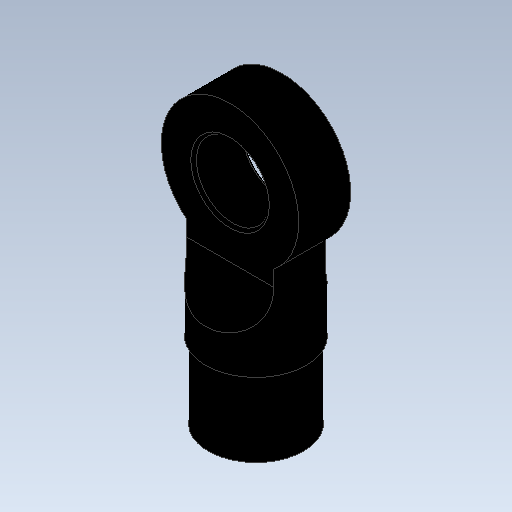
# Autodesk Inventor part: Conexion_superioript
Saved by Autodesk Inventor 2020 (Build 240168000, 168)
## iProperties
Created: 2019-09-21
Part Number: Conexion_superioript
Material: Plástico ABS
Document SubType Name: Modeling
Designer: axelj
Density: 1.06 g/cm^3
Appearance: Anodizado - Negro
Author: axelj
Autodesk Inventor part; units mm, degrees
ref_plane "YZ Plane" through (0, 0, 0) normal (1, 0, 0) x (0, 1, 0)
ref_plane "XZ Plane" through (0, 0, 0) normal (0, 1, 0) x (-1, 0, 0)
ref_plane "XY Plane" through (0, 0, 0) normal (0, 0, 1) x (1, 0, 0)
sketch "Boceto1" plane through (0, 0, 0) normal (0, 1, 0) x (-1, 0, 0)
  circle A0 centre (0, 0) radius 3.4
  dimension "d0" = 6.8
  constraints: 1 centre point, 1 coincident
  measures "d0" diameter of A0
extrude "Extrusión1" add sketch "Boceto1" along normal blind 5.4
sketch "Boceto2" plane through (0, 5.4, 0) normal (0, 1, 0) x (1, 0, 0)
  circle A0 centre (0, 0) radius 3.6
  circle A1 centre (0, 0) radius 3.6
  dimension "d3" = 7.2
  constraints: 2 centre point, 2 coincident
  measures "d3" diameter of A0
extrude "Extrusión2" add sketch "Boceto2" along normal blind 15.3
sketch "Boceto3" plane through (0, 0, 0) normal (0, 0, 1) x (1, 0, 0)
  line L0 (3.4, 5.4) -> (-3.4, 5.4) projected
  line L1 (0, 5.4) -> (0, 10.9)
  line L2 (0, 10.9) -> (0, 15.8)
  circle A0 centre (0, 15.8) radius 4.9
  point P0 (0, 0)
  dimension "d7" = 5.5
  dimension "d8" = 4.9
  constraints: 4 end point, 2 vertical, 1 centre point, 1 coincident, 1 midpoint
  measures "d7" distance of L1.start L1.end
  measures "d8" distance of L1.end L2.end
extrude "Extrusión3" add sketch "Boceto3" along normal blind 1.85 and the other way blind 1.85
sketch "Boceto4" plane through (0, 20.7, 0) normal (0, 1, 0) x (1, 0, 0)
  circle A0 centre (0, 0) radius 3.6 projected
  line L0 (4.9, 1.85) -> (4.9, -1.85) projected
  line L1 (3.0883, -1.85) -> (-3.0883, -1.85)
  line L2 (-4.9, 1.85) -> (-4.9, -1.85) projected
  line L3 (-3.0883, 1.85) -> (-4.9, 1.85) projected
  line L4 (-3.0883, 1.85) -> (3.0883, 1.85)
  line L5 (-3.0883, -1.85) -> (3.0883, -1.85)
  line L6 (3.0883, 1.85) -> (-3.0883, 1.85)
  arc A1 (-3.0883, -1.85) -> (3.0883, -1.85) centre (0, 0) ccw
  arc A2 (3.0883, 1.85) -> (-3.0883, 1.85) centre (0, 0) ccw
  constraints: 8 end point, 6 point on circle, 2 centre point, 2 horizontal, 1 coincident, 1 collinear, 1 parallel
extrude "Extrusión4" cut sketch "Boceto4" against normal blind 9.8 contours L4 A0 | A0 L1
sketch "Boceto5" plane through (0, 0, 1.85) normal (0, 0, 1) x (1, 0, 0)
  arc A0 (-3.0883, 19.6043) -> (-3.0883, 11.9957) centre (0, 15.8) ccw projected
  circle A1 centre (0, 15.8) radius 4.9
  line L0 (-3.6, 19.1242) -> (-3.6, 20.7) projected
  line L1 (-3.6, 19.1242) -> (-3.6, 20.7)
  line L2 (3.6, 20.7) -> (3.0883, 20.7) projected
  line L3 (3.6, 20.7) -> (3.6, 19.1242)
  line L4 (3.6, 19.1242) -> (3.6, 20.7) projected
  line L5 (-3.0883, 20.7) -> (-3.6, 20.7) projected
  line L6 (-3.6, 20.7) -> (3.6, 20.7)
  point P0 (0, 0)
  constraints: 6 end point, 2 collinear, 2 point on circle, 2 point on line, 1 centre point, 1 coincident
extrude "Extrusión5" cut sketch "Boceto5" against normal blind 13 contours A0 L0 L5 L6 A1 | L6 L2 L3 A1
sketch "Boceto6" plane through (0, 0, 0) normal (1, 0, 0) x (0, 1, 0)
  line L0 (10.9, 3.6) -> (10.9, 1.85) projected
  line L1 (10.9, 3.6) -> (10.9, 1.85)
  line L2 (5.4, 3.6) -> (5.4, -3.6) projected
  line L3 (5.4, 3.6) -> (7.8, 3.6)
  line L4 (5.4, 3.6) -> (10.9, 3.6) projected
  arc A0 (7.8, 3.6) -> (10.9, 1.85) centre (10.6815, 5.0837) ccw
  line L5 (0, 0) -> (12.5294, 0)
  line L6 (10.9, -1.85) -> (10.9, -3.6)
  line L7 (5.4, -3.6) -> (10.9, -3.6) projected
  line L8 (10.9, -3.6) -> (10.9, -1.85)
  line L9 (7.8, -3.6) -> (10.9, -3.6)
  arc A1 (10.9, -1.85) -> (7.8, -3.6) centre (10.6815, -5.0837) ccw
  line L10 (7.8, -3.6) -> (10.9, -3.6)
  dimension "d17" = 2.4
  constraints: 14 end point, 6 symmetric about line, 4 point on circle, 2 centre point, 2 collinear, 1 horizontal, 1 point on line, 1 vertical, 1 other
  measures "d17" distance of L2.start L3.end
extrude "Extrusión6" cut sketch "Boceto6" along normal blind 13 and the other way blind 6.5
sketch "Boceto8" plane through (0, 0, 1.85) normal (0, 0, 1) x (1, 0, 0)
  line L0 (3.4, 5.4) -> (-3.4, 5.4) projected
  line L1 (0, 5.4) -> (0, 15.8)
  circle A0 centre (0, 15.8) radius 4.9
  circle A1 centre (0, 15.8) radius 2.6
  point P0 (0, 0)
  dimension "d22" = 10.4
  dimension "d23" = 5.2
  constraints: 2 centre point, 2 coincident, 2 end point, 1 midpoint, 1 vertical
  measures "d22" distance of L1.start L1.end
  measures "d23" diameter of A1
extrude "Extrusión7" cut sketch "Boceto8" against normal blind 13 contours A1
fillet "Empalme1" radius 0.2 1 edges at (-2.6, 15.8, 1.85)
fillet "Empalme2" radius 0.2 1 edges at (-2.6, 15.8, -1.85)
